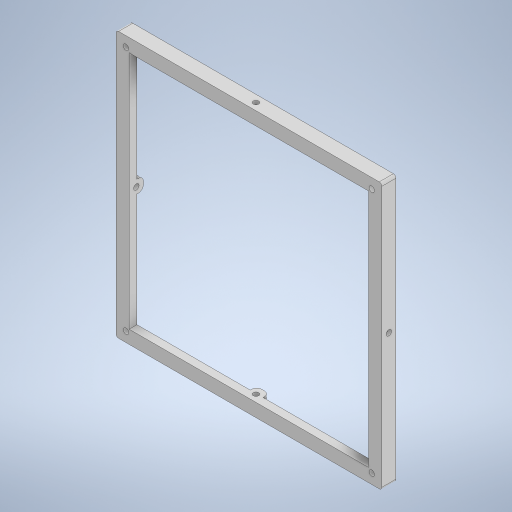
# Autodesk Inventor part: Marco_Tapa
Saved by Autodesk Inventor 2024 (Build 280153000, 153)
## iProperties
Created: 2024-07-18
Part Number: Marco_Tapa
Material: Genérico
Document SubType Name: Modeling
Designer: sergi
Density: 1 g/cm^3
Appearance: Valor por defecto
Author: sergi
Autodesk Inventor part; units mm, degrees
ref_plane "YZ Plane" through (0, 0, 0) normal (1, 0, 0) x (0, 1, 0)
sketch "Boceto1" plane through (0, 0, 0) normal (0, 0, 1) x (1, 0, 0)
  line L0 (-198, 0) -> (0, 0) projected
  line L1 (-198, 0) -> (-198, -2) projected
  line L2 (0, -2) -> (-198, -2) projected
  line L3 (0, 0) -> (0, -2) projected
  line L4 (0, -2) -> (0, -200) projected
  line L5 (0, -2) -> (-2, -2) projected
  line L6 (-2, -200) -> (-2, -2) projected
  line L7 (0, -200) -> (-2, -200) projected
  line L8 (-2.25, -1.75) -> (0.25, -1.75)
  line L9 (0.25, -1.75) -> (0.25, -200.25)
  line L10 (0.25, -200.25) -> (-2.25, -200.25)
  line L11 (-2.25, -200.25) -> (-2.25, -1.75)
  line L12 (-198.25, -2.25) -> (-198.25, 0.25)
  line L13 (-198.25, 0.25) -> (0.25, 0.25)
  line L14 (0.25, 0.25) -> (0.25, -2.25)
  line L15 (0.25, -2.25) -> (-198.25, -2.25)
  line L16 (-200, -198) -> (-200, 0) projected
  line L17 (-200, -198) -> (-198, -198) projected
  line L18 (-198, 0) -> (-198, -198) projected
  line L19 (-200, 0) -> (-198, 0) projected
  line L20 (-2, -200) -> (-200, -200) projected
  line L21 (-2, -200) -> (-2, -198) projected
  line L22 (-200, -198) -> (-2, -198) projected
  line L23 (-200, -200) -> (-200, -198) projected
  line L24 (-200.25, -198) -> (-200.25, 0.25)
  line L25 (-200.25, 0.25) -> (-198, 0.25)
  line L26 (-2, -200.25) -> (-200.25, -200.25)
  line L27 (-200.25, -200.25) -> (-200.25, -198)
  line L28 (-200, -197.75) -> (-1.75, -197.75)
  line L29 (-1.75, -197.75) -> (-1.75, -200)
  line L30 (-197.75, 0) -> (-197.75, -198.25)
  line L31 (-197.75, -198.25) -> (-200, -198.25)
  line L32 (-197.75, -197.75) -> (-2.25, -197.75)
  line L33 (-2.25, -197.75) -> (-2.25, -2.25)
  line L34 (-2.25, -2.25) -> (-197.75, -2.25)
  line L35 (-197.75, -2.25) -> (-197.75, -197.75)
  line L36 (-7.25, -7.25) -> (-7.25, -192.75)
  line L37 (-7.25, -192.75) -> (-192.75, -192.75)
  line L38 (-192.75, -192.75) -> (-192.75, -7.25)
  line L39 (-192.75, -7.25) -> (-7.25, -7.25)
  point P0 (-197.75, -2.25)
  point P1 (-2.25, -197.75)
  point P2 (-2.25, -2.25)
  dimension "d0" = 0.25
  dimension "d1" = 0.25
  dimension "d2" = 0.25
  dimension "d3" = 0.25
  dimension "d4" = 0.25
  dimension "d5" = 0.25
  dimension "d8" = 5
  constraints: 48 end point, 4 parallel, 4 point on line, 2 perpendicular, 1 horizontal, 13 other
  measures "d0" distance between parallel lines of L6 L11
  measures "d1" distance between parallel lines of L2 L15
  measures "d2" distance between parallel lines of L16 L24
  measures "d3" distance between parallel lines of L20 L26
  measures "d4" distance between parallel lines of L22 L28
  measures "d5" distance between parallel lines of L18 L30
  measures "d8" distance between parallel lines of L33 L36
extrude "Extrusión1" add sketch "Boceto1" against normal blind 3 contours L15 L11 L28 L30
sketch "Boceto2" plane through (0, 0, 0) normal (0, 0, 1) x (1, 0, 0)
  line L0 (-197.75, -197.75) -> (-2.25, -197.75) projected
  line L1 (-2.25, -197.75) -> (-2.25, -2.25) projected
  line L2 (-2.25, -2.25) -> (-197.75, -2.25) projected
  line L3 (-197.75, -2.25) -> (-197.75, -197.75) projected
  line L4 (-7.25, -7.25) -> (-7.25, -192.75) projected
  line L5 (-7.25, -192.75) -> (-192.75, -192.75) projected
  line L6 (-192.75, -192.75) -> (-192.75, -7.25) projected
  line L7 (-192.75, -7.25) -> (-7.25, -7.25) projected
  line L8 (0.25, -200.25) -> (-200.25, -200.25)
  line L9 (-200.25, -200.25) -> (-200.25, 0.25)
  line L10 (-200.25, 0.25) -> (0.25, 0.25)
  line L11 (0.25, 0.25) -> (0.25, -200.25)
  line L12 (-203, -203) -> (3, -203)
  line L13 (3, -203) -> (3, 3)
  line L14 (3, 3) -> (-203, 3)
  line L15 (-203, 3) -> (-203, -203)
  point P0 (0, 0)
  dimension "d9" = 2.5
  constraints: 16 end point, 6 other
  measures "d9" distance between parallel lines of L0 L8
extrude "Extrusión2" add sketch "Boceto2" against normal blind 8 contours L15 L14 L13 L12
sketch "Boceto3" plane through (0, 0, 0) normal (0, 0, 1) x (1, 0, 0)
  line L0 (-7, -7) -> (-4, -7) projected
  arc A0 (-4, -7) -> (-7, -4) centre (-7, -7) ccw projected
  line L1 (-197.75, -197.75) -> (-2.25, -197.75) projected
  line L2 (-2.25, -197.75) -> (-2.25, -2.25) projected
  line L3 (-2.25, -2.25) -> (-197.75, -2.25) projected
  line L4 (-197.75, -2.25) -> (-197.75, -197.75) projected
  line L5 (-7.25, -7.25) -> (-7.25, -192.75) projected
  line L6 (-7.25, -192.75) -> (-192.75, -192.75) projected
  line L7 (-192.75, -192.75) -> (-192.75, -7.25) projected
  line L8 (-192.75, -7.25) -> (-7.25, -7.25) projected
  line L9 (3, -203) -> (3, 3) projected
  line L10 (3, 3) -> (-203, 3) projected
  line L11 (-203, 3) -> (-203, -203) projected
  line L12 (-203, -203) -> (3, -203) projected
  line L13 (0.25, -200.25) -> (-200.25, -200.25) projected
  line L14 (-200.25, -200.25) -> (-200.25, 0.25) projected
  line L15 (-200.25, 0.25) -> (0.25, 0.25) projected
  line L16 (0.25, 0.25) -> (0.25, -200.25) projected
  point P0 (0, 0)
extrude "Extrusión3" add sketch "Boceto3" along normal blind 3 contours L4 L3 L2 L1 | L12 L11 L10 L9 | L13 L14 L15 L16
sketch "Boceto4" plane through (0, 0, 3) normal (0, 0, 1) x (1, 0, 0)
  circle A0 centre (-4.75, -4.75) radius 1.5 projected
  circle A1 centre (-195.25, -195.25) radius 1.5 projected
  circle A2 centre (-195.25, -4.75) radius 1.5 projected
  circle A3 centre (-4.75, -4.75) radius 1.5 projected
  circle A4 centre (-4.75, -195.25) radius 1.5 projected
  line L0 (-203, 1) -> (-203, -201) projected
  line L1 (-201, -203) -> (1, -203) projected
  line L2 (3, -201) -> (3, 1) projected
  line L3 (1, 3) -> (-201, 3) projected
  arc A5 (-201, 3) -> (-203, 1) centre (-201, 1) ccw projected
  arc A6 (-203, -201) -> (-201, -203) centre (-201, -201) ccw projected
  arc A7 (1, -203) -> (3, -201) centre (1, -201) ccw projected
  arc A8 (3, 1) -> (1, 3) centre (1, 1) ccw projected
  line L4 (-82, -102) -> (-118, -102) projected
  line L5 (-118, -102) -> (-118, -99) projected
  line L6 (-118, -99) -> (-82, -99) projected
  line L7 (-82, -99) -> (-82, -102) projected
  line L8 (-82, -92) -> (-118, -92) projected
  line L9 (-118, -92) -> (-118, -89) projected
  line L10 (-118, -89) -> (-82, -89) projected
  line L11 (-82, -89) -> (-82, -92) projected
  line L12 (-82, -112) -> (-118, -112) projected
  line L13 (-118, -112) -> (-118, -109) projected
  line L14 (-118, -109) -> (-82, -109) projected
  line L15 (-82, -109) -> (-82, -112) projected
  line L16 (-82, -82) -> (-118, -82) projected
  line L17 (-118, -82) -> (-118, -79) projected
  line L18 (-118, -79) -> (-82, -79) projected
  line L19 (-82, -79) -> (-82, -82) projected
  line L20 (-82, -122) -> (-118, -122) projected
  line L21 (-118, -122) -> (-118, -119) projected
  line L22 (-118, -119) -> (-82, -119) projected
  line L23 (-82, -119) -> (-82, -122) projected
  circle A9 centre (-100, -135) radius 1.5 projected
  circle A10 centre (-100, -65) radius 1.5 projected
  point P0 (0, 0)
hole "Agujero1" at (-195.25, -4.75, 3) at (-195.25, -195.25, 3) at (-4.75, -195.25, 3) at (-4.75, -4.75, 3) direction (0, 0, -1) diameter 4.2 depth 6
ref_plane "Plano de trabajo1" through (-192.75, -100, 3) normal (0, -1, 0) x (1, 0, 0)
sketch "Boceto5" plane through (0, 0, -3) normal (0, 0, -1) x (-1, 0, 0)
  line L0 (2.25, -197.75) -> (197.75, -197.75) projected
  line L1 (197.75, -197.75) -> (197.75, -2.25) projected
  line L2 (197.75, -2.25) -> (2.25, -2.25) projected
  line L3 (2.25, -2.25) -> (2.25, -197.75) projected
  line L4 (7.25, -192.75) -> (7.25, -7.25) projected
  line L5 (7.25, -7.25) -> (192.75, -7.25) projected
  line L6 (192.75, -7.25) -> (192.75, -192.75) projected
  line L7 (192.75, -192.75) -> (7.25, -192.75) projected
  line L8 (197.75, -2.25) -> (2.25, -7.25)
  line L9 (7.25, -7.25) -> (192.75, -7.25) projected
  line L10 (95, -2.25) -> (105, -2.25)
  line L11 (105, -2.25) -> (105, -7.25)
  line L12 (105, -7.25) -> (95, -7.25)
  line L13 (95, -7.25) -> (95, -2.25)
  line L14 (95, -2.25) -> (105, -7.25) construction
  line L15 (105, -2.25) -> (95, -7.25) construction
  point P0 (0, 0)
  point P1 (100, -4.75)
  dimension "d21" = 10
  constraints: 14 end point, 3 midpoint, 3 point on line, 2 parallel, 1 horizontal, 1 perpendicular
  measures "d21" distance of L11.end L12.end
extrude "Extrusión4" add sketch "Boceto5" along normal up to surface (5 mm away) contours L13 L2 L11 L8 | L8 L11 L5 L13
sketch "Boceto6" plane through (-192.75, -7.25, 3) normal (0, -1, 0) x (1, 0, 0)
  line L0 (0, -6) -> (0, 0) projected
  line L1 (87.75, -6) -> (0, -6) projected
  line L2 (87.75, -6) -> (87.75, -11) projected
  line L3 (87.75, -11) -> (97.75, -11) projected
  line L4 (97.75, -6) -> (97.75, -11) projected
  line L5 (185.5, -6) -> (97.75, -6) projected
  line L6 (185.5, 0) -> (185.5, -6) projected
  line L7 (0, 0) -> (185.5, 0) projected
  line L8 (87.75, -11) -> (97.75, -11)
  line L9 (97.75, -11) -> (97.75, 0)
  line L10 (97.75, 0) -> (87.75, 0)
  line L11 (87.75, 0) -> (87.75, -11)
  line L12 (87.75, -6) -> (87.75, -11) projected
  line L13 (87.75, -11) -> (97.75, 0)
  circle A0 centre (92.75, -5.5) radius 2.1
  point P0 (192.75, -3)
  dimension "d24" = 4.2
  constraints: 10 end point, 2 parallel, 1 centre point, 1 horizontal, 1 midpoint, 1 perpendicular, 1 point on line
  measures "d24" diameter of A0
hole "Agujero2" at (-100, -7.25, -2.5) direction (0, 1, 0) diameter 4.2 end through all
fillet "Empalme1" radius 4 2 edges at (-105, -4.75, -8) (-95, -4.75, -8)
mirror "Simetría1" about plane through (-192.75, -100, 3) normal (0, -1, 0) of "Extrusión4", "Agujero2", "Empalme1"
ref_plane "Plano de trabajo2" through (-192.75, -192.75, 0) normal (-0.7071068, 0.7071068, 0) x (0, 0, 1)
mirror "Simetría2" about plane through (-192.75, -192.75, 0) normal (-0.7071068, 0.7071068, 0) of "Extrusión4", "Agujero2", "Empalme1", "Simetría1"
fillet "Empalme2" radius 2 4 edges at (-203, 3, -2.5) (-203, -203, -2.5) (3, -203, -2.5) (3, 3, -2.5)
fillet "Empalme3" radius 2 28 edges at (-151.375, -2.25, -3) (-48.625, -2.25, -3) (-2.25, -48.625, -3) (-2.25, -151.375, -3) (-48.625, -197.75, -3) (-151.375, -197.75, -3) (-197.75, -48.625, -3) (-197.75, -151.375, -3) (-197.75, -95, -3.5) (-197.75, -100, -8) (-197.75, -103.8284, -6.8284) (-197.75, -105, -3.5) (-197.75, -96.1716, -6.8284) (-103.8284, -2.25, -6.8284) (-105, -2.25, -3.5) (-96.1716, -2.25, -6.8284) (-95, -2.25, -3.5) (-100, -2.25, -8) (-2.25, -100, -8) (-2.25, -103.8284, -6.8284) (-2.25, -105, -3.5) (-2.25, -95, -3.5) (-2.25, -96.1716, -6.8284) (-105, -197.75, -3.5) (-100, -197.75, -8) (-96.1716, -197.75, -6.8284) (-95, -197.75, -3.5) (-103.8284, -197.75, -6.8284)
